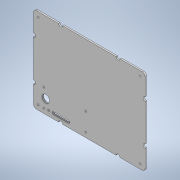
# Autodesk Inventor part: AcrylicCover
Saved by Autodesk Inventor 2022 (Build 260153000, 153)
## iProperties
Created: 2021-11-11
Part Number: AcrylicCover
Material: Generic
Document SubType Name: Modeling
Designer: Viktor
Density: 1 g/cm^3
Appearance: Default
Author: Viktor
Autodesk Inventor part; units mm, degrees
ref_plane "YZ Plane" through (0, 0, 0) normal (1, 0, 0) x (0, 1, 0)
ref_plane "XZ Plane" through (0, 0, 0) normal (0, 1, 0) x (-1, 0, 0)
ref_plane "XY Plane" through (0, 0, 0) normal (0, 0, 1) x (1, 0, 0)
sketch "Sketch1" plane through (0, 0, 0) normal (0, 0, 1) x (1, 0, 0)
  line L0 (-117.5, -90) -> (117.5, -90)
  line L1 (117.5, -90) -> (117.5, 90)
  line L2 (117.5, 90) -> (-117.5, 90)
  line L3 (-117.5, 90) -> (-117.5, -90)
  line L4 (-117.5, -90) -> (117.5, 90) construction
  line L5 (117.5, -90) -> (-117.5, 90) construction
  point P0 (0, 0)
  dimension "d0" = 235
  dimension "d1" = 180
  constraints: 12 end point, 2 midpoint, 2 parallel, 1 horizontal, 1 perpendicular
  measures "d0" distance between parallel lines of L1 L3
  measures "d1" distance between parallel lines of L0 L2
extrude "Extrusion1" add sketch "Sketch1" along normal blind 3
fillet "Fillet1" radius 6 4 edges at (117.5, -90, 1.5) (-117.5, -90, 1.5) (-117.5, 90, 1.5) (117.5, 90, 1.5)
sketch "Sketch2" plane through (0, 0, 3) normal (0, 0, 1) x (1, 0, 0)
  line L0 (-111.5, -90) -> (111.5, -90) construction
  arc A0 (-117.5, -84) -> (-111.5, -90) centre (-111.5, -84) ccw projected
  line L1 (-117.5, 84) -> (-117.5, -84) projected
  arc A1 (-111.5, 90) -> (-117.5, 84) centre (-111.5, 84) ccw projected
  line L2 (111.5, 90) -> (-111.5, 90) projected
  arc A2 (117.5, 84) -> (111.5, 90) centre (111.5, 84) ccw projected
  line L3 (117.5, -84) -> (117.5, 84) construction
  arc A3 (111.5, -90) -> (117.5, -84) centre (111.5, -84) ccw construction
  line L4 (-111.5, -90) -> (111.5, -90) projected
  circle A4 centre (60.5, -90) radius 4.125
  line L5 (117.5, -84) -> (117.5, 84) projected
  circle A5 centre (117.5, -43) radius 4.125
  line L6 (-247.3162, 0) -> (250.1985, 0) projected
  line L7 (0, 198.3162) -> (0, -201.1985) projected
  arc A6 (-117.5, -84) -> (-111.5, -90) centre (-111.5, -84) ccw construction
  circle A7 centre (-60.5, -90) radius 4.125
  circle A8 centre (-117.5, -43) radius 4.125
  line L8 (-111.5, 90) -> (111.5, 90) construction
  arc A9 (-111.5, 90) -> (-117.5, 84) centre (-111.5, 84) ccw
  arc A10 (117.5, 84) -> (111.5, 90) centre (111.5, 84) ccw construction
  line L9 (-111.5, 90) -> (111.5, 90)
  circle A11 centre (60.5, 90) radius 4.125
  circle A12 centre (117.5, 43) radius 4.125
  circle A13 centre (-117.5, 43) radius 4.125
  arc A14 (-111.5, 90) -> (-117.5, 84) centre (-111.5, 84) ccw construction
  circle A15 centre (-60.5, 90) radius 4.125
  point P0 (0, 0)
  point P1 (-56.375, -90)
  point P2 (-64.625, -90)
  point P3 (-117.5, -38.875)
  point P4 (-117.5, -47.125)
  point P5 (-117.5, 47.125)
  point P6 (-117.5, 38.875)
  point P7 (-64.625, 90)
  point P8 (-56.375, 90)
  point P9 (56.375, 90)
  point P10 (64.625, 90)
  point P11 (117.5, 47.125)
  point P12 (117.5, 38.875)
  point P13 (117.5, -38.875)
  point P14 (117.5, -47.125)
  point P15 (64.625, -90)
  point P16 (56.375, -90)
  dimension "d5" = 8.25
  dimension "d6" = 8.25
  dimension "d7" = 57
  dimension "d8" = 47
  constraints: 12 centre point, 10 symmetric about line, 8 point on circle, 4 end point, 3 point on line, 10 other
  measures "d5" diameter of A4
  measures "d6" diameter of A5
  measures "d7" distance from line of L3 A4.centre
  measures "d8" distance from line of L0 A5.centre
extrude "Extrusion2" cut sketch "Sketch2" against normal through all contours L1 A8 | A7 L4 | L1 A13 | A12 L5 | L2 A11 | A15 L2 | A4 L4 | A5 L5 picked at (-116.0461, -41.7888) picked at (-60.3343, -88.635) picked at (-116.0461, 44.2112) picked at (115.6202, 41.8533) picked at (60.6657, 88.635) picked at (-60.3343, 88.635) picked at (60.6657, -88.635) picked at (115.6202, -44.1467)
sketch "Sketch3" plane through (0, 0, 3) normal (0, 0, 1) x (1, 0, 0)
  circle A0 centre (107.5, -80) radius 1.75
  line L0 (117.5, -38.875) -> (117.5, 38.875) projected
  line L1 (64.625, -90) -> (111.5, -90) construction
  line L2 (0, 126) -> (0, -126) projected
  line L3 (-164.5, 0) -> (164.5, 0) projected
  circle A1 centre (-107.5, -80) radius 1.75
  circle A2 centre (107.5, 80) radius 1.75
  line L4 (64.625, 90) -> (111.5, 90) construction
  circle A3 centre (-107.5, 80) radius 1.75
  point P0 (0, 0)
  point P1 (-111.5, -90)
  point P2 (-111.5, 90)
  dimension "d11" = 3.5
  dimension "d12" = 10
  dimension "d13" = 10
  constraints: 7 symmetric about line, 4 centre point, 2 end point, 3 other
  measures "d11" diameter of A0
  measures "d12" distance from line of L0 A0.centre
  measures "d13" distance from line of L1 A0.centre
extrude "Extrusion3" cut sketch "Sketch3" against normal blind 10
sketch "Sketch4" plane through (0, 0, 3) normal (0, 0, 1) x (1, 0, 0)
  circle A0 centre (-91.5, -61) radius 8
  circle A1 centre (-85.5, -79) radius 2
  line L0 (-43.5, -79) -> (-75.5, -79) construction
  line L1 (-43.5, -76.5) -> (-75.5, -76.5)
  line L2 (-75.5, -81.5) -> (-43.5, -81.5)
  arc A2 (-43.5, -81.5) -> (-43.5, -76.5) centre (-43.5, -79) ccw
  arc A3 (-75.5, -76.5) -> (-75.5, -81.5) centre (-75.5, -79) ccw
  circle A4 centre (-95.5, -80) radius 1.5
  line L3 (-23, -61) -> (-106, -61) construction
  line L4 (-51.5, -84) -> (-51.5, -34) construction
  circle A5 centre (-7.5, -80) radius 1.5
  circle A6 centre (-95.5, -42) radius 1.5
  circle A7 centre (-7.5, -42) radius 1.5
  line L5 (-111.5, -90) -> (-64.625, -90) projected
  line L6 (-117.5, -47.125) -> (-117.5, -84) projected
  point P0 (0, 0)
  point P1 (-59.5, -79)
  dimension "d16" = 2.5
  dimension "d17" = 16
  dimension "d18" = 4
  dimension "d19" = 10
  dimension "d20" = 32
  dimension "d21" = 6
  dimension "d22" = 18
  dimension "d23" = 34
  dimension "d24" = 18
  dimension "d25" = 44
  dimension "d26" = 19
  dimension "d27" = 3
  dimension "d28" = 10
  dimension "d29" = 22
  dimension "d30" = 0
  constraints: 12 end point, 8 centre point, 4 point on circle, 4 tangent, 3 symmetric about line, 2 horizontal, 1 midpoint, 1 parallel, 1 vertical, 3 other
  measures "d16" radius of A3
  measures "d17" diameter of A0
  measures "d18" diameter of A1
  measures "d19" distance of L0.end A1.centre
  measures "d20" distance of L0.end L0.start
  measures "d21" horizontal distance of A0.centre A1.centre
  measures "d22" vertical distance of A1.centre A0.centre
  measures "d23" distance from line of L4 A1.centre
  measures "d24" distance from line of A1.centre L3
  measures "d25" distance from line of L4 A4.centre
  measures "d26" distance from line of L3 A4.centre
  measures "d27" diameter of A4
  measures "d28" distance from line of L5 A4.centre
  measures "d29" distance from line of L6 A4.centre
  measures "d30" vertical distance of A1.centre point (-59.5, -79)
extrude "Extrusion4" cut sketch "Sketch4" against normal through all
equation "\"d6\" = d5"
equation "\"d13\" = d12"
body "Solid1"
